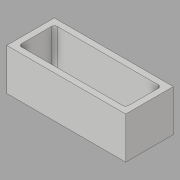
# Autodesk Inventor part: Electronics Box
Saved by Autodesk Inventor 2017 (Build 210142000, 142)
## iProperties
Created: 2017-02-16
Part Number: Electronics Box
Material: Generic
Document SubType Name: Modeling
Designer: qupec
Density: 1 g/cm^3
Appearance: Default
Author: qupec
Autodesk Inventor part; units mm, degrees
ref_plane "YZ Plane" through (0, 0, 0) normal (1, 0, 0) x (0, 1, 0)
ref_plane "XZ Plane" through (0, 0, 0) normal (0, 1, 0) x (-1, 0, 0)
ref_plane "XY Plane" through (0, 0, 0) normal (0, 0, 1) x (1, 0, 0)
sketch "Sketch1" plane through (0, 0, 0) normal (0, 1, 0) x (-1, 0, 0)
  line L0 (63.5, 25.4) -> (-63.5, 25.4)
  line L1 (-63.5, 25.4) -> (-63.5, -25.4)
  line L2 (-63.5, -25.4) -> (63.5, -25.4)
  line L3 (63.5, -25.4) -> (63.5, 25.4)
  point P0 (0, 0)
  dimension "d0" = 50.8
  dimension "d1" = 25.4
  dimension "d2" = 63.5
  dimension "d3" = 127
  constraints: 8 end point, 2 parallel, 1 horizontal, 1 perpendicular
  measures "d0" distance between parallel lines of L2 L0
  measures "d1" distance from line of point (0, 0) L0
  measures "d2" distance from line of point (0, 0) L1
  measures "d3" distance of L0.start L0.end
extrude "Extrusion1" add sketch "Sketch1" along normal blind 6.35
sketch "Sketch2" plane through (0, 6.35, 0) normal (0, 1, 0) x (1, 0, 0)
  line L0 (-57.15, -19.05) -> (57.15, -19.05)
  line L1 (57.15, -19.05) -> (57.15, 19.05)
  line L2 (57.15, 19.05) -> (-57.15, 19.05)
  line L3 (-57.15, 19.05) -> (-57.15, -19.05)
  line L4 (-63.5, -25.4) -> (63.5, -25.4) projected
  line L5 (63.5, -25.4) -> (63.5, 25.4) projected
  line L6 (63.5, 25.4) -> (-63.5, 25.4) projected
  line L7 (-63.5, 25.4) -> (-63.5, -25.4) projected
  point P0 (0, 0)
  dimension "d6" = 6.35
  dimension "d7" = 6.35
  dimension "d8" = 6.35
  dimension "d9" = 6.35
  constraints: 8 end point, 2 parallel, 1 horizontal, 1 perpendicular
  measures "d6" distance between parallel lines of L7 L3
  measures "d7" distance between parallel lines of L4 L0
  measures "d8" distance between parallel lines of L5 L1
  measures "d9" distance between parallel lines of L6 L2
extrude "Extrusion2" add sketch "Sketch2" along normal blind 38.1
fillet "Fillet1" radius 3.175 4 edges at (-57.15, 25.4, -19.05) (57.15, 25.4, -19.05) (57.15, 25.4, 19.05) (-57.15, 25.4, 19.05)
equation "\"d1\" = 0.5 * d0"
equation "\"d2\" = 0.5 * d3"
equation "\"d7\" = d6"
equation "\"d8\" = d6"
equation "\"d9\" = d6"
body "Solid1"
